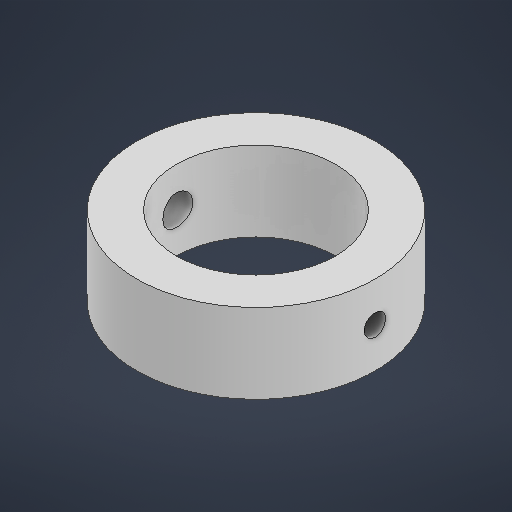
# Autodesk Inventor part: taper pin
Saved by Autodesk Inventor 2026.3 (Build 303398000, 398)
## iProperties
Created: 2026-07-15
Part Number: taper pin
Material: Generic
Document SubType Name: Modeling
Designer: User
Density: 1 g/cm^3
Appearance: Default
Author: User
Autodesk Inventor part; units mm, degrees
ref_plane "YZ Plane" through (0, 0, 0) normal (1, 0, 0) x (0, 1, 0)
ref_plane "XZ Plane" through (0, 0, 0) normal (0, 1, 0) x (-1, 0, 0)
ref_plane "XY Plane" through (0, 0, 0) normal (0, 0, 1) x (1, 0, 0)
sketch "Sketch1" plane through (0, 0, 0) normal (0, 1, 0) x (-1, 0, 0)
  circle A0 centre (0, 0) radius 22.5
  circle A1 centre (0, 0) radius 15
  dimension "d0" = 45
  dimension "d1" = 30
  constraints: 2 centre point, 2 coincident
  measures "d0" diameter of A0
  measures "d1" diameter of A1
extrude "Extrusion1" add sketch "Sketch1" along normal mid plane 15
sketch "Sketch2" plane through (0, 0, 0) normal (0, 0, 1) x (1, 0, 0)
  line L0 (-22.5, -7.5) -> (-22.5, 7.5) projected
  line L1 (-22.5, 0) -> (22.5, 0)
  line L2 (22.5, -7.5) -> (22.5, 7.5) projected
  line L3 (-22.5, 0) -> (-22.5, 3)
  line L4 (22.5, 0) -> (22.5, 2)
  line L5 (22.5, 2) -> (-22.5, 3)
  point P0 (0, 0)
  dimension "d4" = 3
  dimension "d5" = 2
  constraints: 8 end point, 2 midpoint, 2 point on line
  measures "d4" distance of L1.start L3.end
  measures "d5" distance of L1.end L4.end
revolve "Revolution1" cut sketch "Sketch2" angle 360 about axis through (-22.5, 0, 0) along (1, 0, 0)
body "Solid1"
